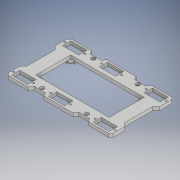
# Autodesk Inventor part: BODY_TOP
Saved by Autodesk Inventor 2017.3 (Build 213256000, 256)
## iProperties
Created: 2017-09-24
Part Number: BODY_TOP
Material: Generic
Document SubType Name: Modeling
Designer: Alexander Miller
Density: 1 g/cm^3
Appearance: Default
body_C_Top: 5,000 mm
Author: Alexander Miller
Autodesk Inventor part; units mm, degrees
ref_plane "YZ Plane" through (0, 0, 0) normal (1, 0, 0) x (0, 1, 0)
ref_plane "XZ Plane" through (0, 0, 0) normal (0, 1, 0) x (-1, 0, 0)
ref_plane "XY Plane" through (0, 0, 0) normal (0, 0, 1) x (1, 0, 0)
sketch "Sketch1" plane through (0, 0, 0) normal (0, 1, 0) x (-1, 0, 0)
  line L0 (45, -75) -> (-45, -75)
  line L1 (-45, -75) -> (-45, 75)
  line L2 (-45, 75) -> (45, 75)
  line L3 (45, 75) -> (45, -75)
  point P0 (0, 0)
  point P1 (0, -75)
  point P2 (45, 0)
  dimension "d0" = 90
  dimension "d1" = 150
  constraints: 8 end point, 2 midpoint, 2 parallel, 1 horizontal, 1 horizontal alignment, 1 perpendicular, 1 vertical alignment
  measures "d0" distance of L0.start L0.end
  measures "d1" distance of L2.end L0.start
extrude "Extrusion1" add sketch "Sketch1" along normal blind 5
sketch "Sketch2" plane through (0, 5, 0) normal (0, 1, 0) x (1, 0, 0)
  line L0 (-42.5, 69.75) -> (-30.5, 69.75)
  line L1 (-30.5, 69.75) -> (-30.5, 46.75)
  line L2 (-30.5, 46.75) -> (-42.5, 46.75)
  line L3 (-42.5, 46.75) -> (-42.5, 69.75)
  line L4 (-42.5, 17) -> (-30.5, 17)
  line L5 (-30.5, 17) -> (-30.5, -6)
  line L6 (-30.5, -6) -> (-42.5, -6)
  line L7 (-42.5, -6) -> (-42.5, 17)
  line L8 (-42.5, -46.75) -> (-30.5, -46.75)
  line L9 (-30.5, -46.75) -> (-30.5, -69.75)
  line L10 (-30.5, -69.75) -> (-42.5, -69.75)
  line L11 (-42.5, -69.75) -> (-42.5, -46.75)
  line L12 (-45, 75) -> (-45, -75) projected
  line L13 (45, 75) -> (-45, 75) projected
  line L14 (-45, -75) -> (45, -75) projected
  circle A0 centre (-36.5, 0) radius 6 construction
  circle A1 centre (-36.5, 72.5) radius 1.25
  circle A2 centre (-36.5, 44) radius 1.25
  circle A3 centre (-36.5, 19.75) radius 1.25
  circle A4 centre (-36.5, -8.75) radius 1.25
  circle A5 centre (-36.5, -44) radius 1.25
  circle A6 centre (-36.5, -72.5) radius 1.25
  line L15 (0, 105) -> (0, -105) construction
  line L16 (42.5, 69.75) -> (30.5, 69.75)
  line L17 (30.5, 69.75) -> (30.5, 46.75)
  line L18 (30.5, 46.75) -> (42.5, 46.75)
  line L19 (42.5, 46.75) -> (42.5, 69.75)
  line L20 (42.5, 17) -> (30.5, 17)
  line L21 (30.5, 17) -> (30.5, -6)
  line L22 (30.5, -6) -> (42.5, -6)
  line L23 (42.5, -6) -> (42.5, 17)
  line L24 (42.5, -46.75) -> (30.5, -46.75)
  line L25 (30.5, -46.75) -> (30.5, -69.75)
  line L26 (30.5, -69.75) -> (42.5, -69.75)
  line L27 (42.5, -69.75) -> (42.5, -46.75)
  circle A7 centre (36.5, 72.5) radius 1.25
  circle A8 centre (36.5, 44) radius 1.25
  circle A9 centre (36.5, 19.75) radius 1.25
  circle A10 centre (36.5, -8.75) radius 1.25
  circle A11 centre (36.5, -44) radius 1.25
  circle A12 centre (36.5, -72.5) radius 1.25
  point P0 (0, 0)
  point P1 (-36.5, 46.75)
  point P2 (-36.5, 17)
  point P3 (-36.5, -6)
  point P4 (-36.5, -46.75)
  point P5 (-36.5, 69.75)
  point P6 (-36.5, -69.75)
  dimension "d4" = 2.5
  dimension "d5" = 5.25
  dimension "d6" = 23
  dimension "d7" = 12
  dimension "d8" = 5.25
  dimension "d9" = 2.5
  dimension "d10" = 1.5
  dimension "d11" = 1.5
  dimension "d12" = 1.5
  dimension "d13" = 1.5
  dimension "d14" = 1.5
  dimension "d15" = 1.5
  constraints: 48 end point, 18 symmetric about line, 13 centre point, 8 vertical alignment, 6 midpoint, 6 parallel, 5 equal radius, 3 equal length, 3 horizontal, 3 perpendicular, 3 tangent, 2 point on line, 1 horizontal alignment, 6 other
  measures "d4" distance between parallel lines of L3 L12
  measures "d5" distance between parallel lines of L13 L0
  measures "d6" distance of L2.end L0.start
  measures "d7" distance of L0.start L0.end
  measures "d8" distance between parallel lines of L14 L10
  measures "d9" diameter of A1
  measures "d10" distance edge to line of A1 L0
  measures "d11" distance edge to line of A2 L2
  measures "d12" distance edge to line of A3 L4
  measures "d13" distance edge to line of A4 L6
  measures "d14" distance edge to line of A5 L8
  measures "d15" distance edge to line of A6 L10
extrude "Extrusion2" cut sketch "Sketch2" against normal through all
sketch "Sketch3" plane through (0, 5, 0) normal (0, 1, 0) x (1, 0, 0)
  line L0 (45, 42.875) -> (40, 39.875)
  line L1 (40, 39.875) -> (40, 23.875)
  line L2 (45, -75) -> (45, 75) projected
  line L3 (40, 23.875) -> (45, 20.875)
  line L4 (45, 20.875) -> (45, 42.875)
  line L5 (42.5, 46.75) -> (30.5, 46.75) projected
  line L6 (36.5, 46.75) -> (36.5, 17) construction
  line L7 (30.5, 17) -> (42.5, 17) projected
  line L8 (-63, 0) -> (63, 0) projected
  line L9 (0, 105) -> (0, -105) projected
  line L10 (45, -42.875) -> (40, -39.875)
  line L11 (40, -39.875) -> (40, -23.875)
  line L12 (40, -23.875) -> (45, -20.875)
  line L13 (45, -20.875) -> (45, -42.875)
  line L14 (-45, 42.875) -> (-40, 39.875)
  line L15 (-40, 39.875) -> (-40, 23.875)
  line L16 (-40, 23.875) -> (-45, 20.875)
  line L17 (-45, 20.875) -> (-45, 42.875)
  line L18 (-45, -42.875) -> (-40, -39.875)
  line L19 (-40, -39.875) -> (-40, -23.875)
  line L20 (-40, -23.875) -> (-45, -20.875)
  line L21 (-45, -20.875) -> (-45, -42.875)
  line L22 (25, 75) -> (-25, 75)
  line L23 (-25, 75) -> (-20, 70)
  line L24 (-20, 70) -> (20, 70)
  line L25 (20, 70) -> (25, 75)
  line L26 (45, 75) -> (-45, 75) projected
  line L27 (25, -75) -> (-25, -75)
  line L28 (-25, -75) -> (-20, -70)
  line L29 (-20, -70) -> (20, -70)
  line L30 (20, -70) -> (25, -75)
  point P0 (0, 0)
  point P1 (45, 31.875)
  point P2 (40, 31.875)
  point P3 (36.5, 31.875)
  point P4 (0, 70)
  point P5 (0, 75)
  dimension "d38" = 16
  dimension "d39" = 22
  dimension "d40" = 40
  dimension "d41" = 50
  dimension "d42" = 5
  dimension "d43" = 5
  constraints: 50 end point, 16 symmetric about line, 7 midpoint, 3 parallel, 2 collinear, 2 equal length, 2 horizontal alignment, 2 vertical alignment, 1 perpendicular
  measures "d38" distance of L0.end L1.end
  measures "d39" distance of L3.end L0.start
  measures "d40" distance of L23.end L24.end
  measures "d41" distance of L22.start L22.end
  measures "d42" distance between parallel lines of L26 L24
  measures "d43" distance between parallel lines of L1 L4
extrude "Extrusion3" cut sketch "Sketch3" against normal through all contours L2 L3 L1 L0 | L2 L10 L11 L12 | L29 L30 L27 L9 | L9 L27 L28 L29 | L25 L24 L9 L22 | L9 L24 L23 L22 | L14 L15 L16 L17 | L21 L20 L19 L18
chamfer "Chamfer1" distance 3 angle 45 4 edges at (45, 2.5, 75) (-45, 2.5, 75) (-45, 2.5, -75) (45, 2.5, -75)
sketch "Sketch4" plane through (0, 5, 0) normal (0, 1, 0) x (1, 0, 0)
  line L0 (25, 52.5) -> (-25, 52.5)
  line L1 (-25, 52.5) -> (-25, -52.5)
  line L2 (-25, -52.5) -> (25, -52.5)
  line L3 (25, -52.5) -> (25, 52.5)
  point P0 (0, 0)
  point P1 (25, 0)
  point P2 (0, 52.5)
  dimension "d23" = 105
  dimension "d24" = 50
  constraints: 8 end point, 2 midpoint, 2 parallel, 1 horizontal, 1 horizontal alignment, 1 perpendicular, 1 vertical alignment
  measures "d23" distance of L2.end L0.start
  measures "d24" distance of L1.end L2.end
extrude "Extrusion4" cut sketch "Sketch4" against normal blind 5
sketch "Sketch7" plane through (0, 5, 0) normal (0, 1, 0) x (1, 0, 0)
  circle A0 centre (36.5, 31.875) radius 1.675
  line L0 (-63, 0) -> (63, 0) projected
  line L1 (0, 105) -> (0, -105) projected
  line L2 (40, 23.875) -> (40, 39.875) projected
  line L3 (30.5, 17) -> (42.5, 17) projected
  circle A1 centre (36.5, -31.875) radius 1.675
  circle A2 centre (-36.5, 31.875) radius 1.675
  circle A3 centre (-36.5, -31.875) radius 1.675
  point P0 (0, 0)
  point P1 (40, 31.875)
  point P2 (36.5, 17)
  dimension "d44" = 3.35
  constraints: 4 centre point, 3 symmetric about line, 2 midpoint, 1 horizontal alignment, 1 vertical alignment, 3 other
  measures "d44" diameter of A0
extrude "Extrusion7" cut sketch "Sketch7" against normal through all
sketch "Sketch8" plane through (0, 0, 0) normal (0, -1, 0) x (1, 0, 0)
  line L0 (-38.675, -46.175) -> (-34.325, -46.175)
  line L1 (-34.325, -46.175) -> (-34.325, -41.825)
  line L2 (-34.325, -41.825) -> (-38.675, -41.825)
  line L3 (-38.675, -41.825) -> (-38.675, -46.175)
  line L4 (-38.675, -74.675) -> (-34.325, -74.675)
  line L5 (-34.325, -74.675) -> (-34.325, -70.325)
  line L6 (-34.325, -70.325) -> (-38.675, -70.325)
  line L7 (-38.675, -70.325) -> (-38.675, -74.675)
  line L8 (-38.675, -21.925) -> (-34.325, -21.925)
  line L9 (-34.325, -21.925) -> (-34.325, -17.575)
  line L10 (-34.325, -17.575) -> (-38.675, -17.575)
  line L11 (-38.675, -17.575) -> (-38.675, -21.925)
  line L12 (-38.675, 6.575) -> (-34.325, 6.575)
  line L13 (-34.325, 6.575) -> (-34.325, 10.925)
  line L14 (-34.325, 10.925) -> (-38.675, 10.925)
  line L15 (-38.675, 10.925) -> (-38.675, 6.575)
  line L16 (-38.675, 41.825) -> (-34.325, 41.825)
  line L17 (-34.325, 41.825) -> (-34.325, 46.175)
  line L18 (-34.325, 46.175) -> (-38.675, 46.175)
  line L19 (-38.675, 46.175) -> (-38.675, 41.825)
  line L20 (-34.325, 70.325) -> (-38.675, 70.325)
  line L21 (-38.675, 70.325) -> (-38.675, 74.675)
  line L22 (-38.675, 74.675) -> (-34.325, 74.675)
  line L23 (-34.325, 74.675) -> (-34.325, 70.325)
  circle A0 centre (-36.5, -72.5) radius 1.25 projected
  circle A1 centre (-36.5, -44) radius 1.25 projected
  circle A2 centre (-36.5, -19.75) radius 1.25 projected
  circle A3 centre (-36.5, 8.75) radius 1.25 projected
  circle A4 centre (-36.5, 44) radius 1.25 projected
  circle A5 centre (-36.5, 72.5) radius 1.25 projected
  line L24 (0, -105) -> (0, 105) projected
  line L25 (38.675, -46.175) -> (34.325, -46.175)
  line L26 (34.325, -46.175) -> (34.325, -41.825)
  line L27 (34.325, -41.825) -> (38.675, -41.825)
  line L28 (38.675, -41.825) -> (38.675, -46.175)
  line L29 (38.675, -74.675) -> (34.325, -74.675)
  line L30 (34.325, -74.675) -> (34.325, -70.325)
  line L31 (34.325, -70.325) -> (38.675, -70.325)
  line L32 (38.675, -70.325) -> (38.675, -74.675)
  line L33 (38.675, -21.925) -> (34.325, -21.925)
  line L34 (34.325, -21.925) -> (34.325, -17.575)
  line L35 (34.325, -17.575) -> (38.675, -17.575)
  line L36 (38.675, -17.575) -> (38.675, -21.925)
  line L37 (38.675, 6.575) -> (34.325, 6.575)
  line L38 (34.325, 6.575) -> (34.325, 10.925)
  line L39 (34.325, 10.925) -> (38.675, 10.925)
  line L40 (38.675, 10.925) -> (38.675, 6.575)
  line L41 (38.675, 41.825) -> (34.325, 41.825)
  line L42 (34.325, 41.825) -> (34.325, 46.175)
  line L43 (34.325, 46.175) -> (38.675, 46.175)
  line L44 (38.675, 46.175) -> (38.675, 41.825)
  line L45 (34.325, 70.325) -> (38.675, 70.325)
  line L46 (38.675, 70.325) -> (38.675, 74.675)
  line L47 (38.675, 74.675) -> (34.325, 74.675)
  line L48 (34.325, 74.675) -> (34.325, 70.325)
  point P0 (0, 0)
  point P1 (-36.5, -74.675)
  point P2 (-36.5, -46.175)
  point P3 (-36.5, -41.825)
  point P4 (-36.5, -21.925)
  point P5 (-36.5, -17.575)
  point P6 (-36.5, 6.575)
  point P7 (-36.5, 10.925)
  point P8 (-36.5, 41.825)
  point P9 (-36.5, 46.175)
  point P10 (-36.5, 70.325)
  point P11 (-38.675, -72.5)
  point P12 (-38.675, -44)
  point P13 (-38.675, -19.75)
  point P14 (-38.675, 8.75)
  point P15 (-38.675, 72.5)
  point P16 (-38.675, 44)
  dimension "d47" = 4.35
  constraints: 96 end point, 24 symmetric about line, 16 midpoint, 12 parallel, 11 equal length, 6 horizontal, 6 horizontal alignment, 6 perpendicular, 6 vertical alignment, 2 point on line
  measures "d47" distance of L6.end L4.start
extrude "Extrusion8" cut sketch "Sketch8" against normal blind 1.725
sketch "Sketch9" plane through (0, 5, 0) normal (0, 1, 0) x (1, 0, 0)
  circle A0 centre (36.5, 31.875) radius 2.925
  circle A1 centre (36.5, -31.875) radius 2.925
  circle A2 centre (-36.5, -31.875) radius 2.925
  circle A3 centre (-36.5, 31.875) radius 2.925
  circle A4 centre (36.5, 31.875) radius 1.675 projected
  circle A5 centre (36.5, -31.875) radius 1.675 projected
  circle A6 centre (-36.5, -31.875) radius 1.675 projected
  circle A7 centre (-36.5, 31.875) radius 1.675 projected
  point P0 (0, 0)
  dimension "d50" = 5.85
  constraints: 4 centre point, 4 concentric, 3 equal radius
  measures "d50" diameter of A0
extrude "Extrusion9" cut sketch "Sketch9" against normal blind 3
sketch "Sketch11" plane through (0, 0, 0) normal (0, -1, 0) x (1, 0, 0)
  line L0 (-19.65, -57.5) -> (-30, -57.5)
  line L1 (-30, -57.5) -> (-30, -47.15)
  line L2 (-30, -47.15) -> (-19.65, -47.15)
  line L3 (-19.65, -47.15) -> (-19.65, -57.5)
  line L4 (-30, 47.15) -> (-19.65, 47.15)
  line L5 (-19.65, 47.15) -> (-19.65, 57.5)
  line L6 (-19.65, 57.5) -> (-30, 57.5)
  line L7 (-30, 57.5) -> (-30, 47.15)
  line L8 (19.65, 57.5) -> (30, 57.5)
  line L9 (30, 57.5) -> (30, 47.15)
  line L10 (30, 47.15) -> (19.65, 47.15)
  line L11 (19.65, 47.15) -> (19.65, 57.5)
  line L12 (19.65, -57.5) -> (30, -57.5)
  line L13 (30, -57.5) -> (30, -47.15)
  line L14 (30, -47.15) -> (19.65, -47.15)
  line L15 (19.65, -47.15) -> (19.65, -57.5)
  line L16 (-25, -52.5) -> (-25, 52.5) projected
  line L17 (25, -52.5) -> (-25, -52.5) projected
  line L18 (-25, 52.5) -> (25, 52.5) projected
  line L19 (25, 52.5) -> (25, -52.5) projected
  point P0 (0, 0)
  point P1 (-19.65, -52.325)
  point P2 (19.65, -52.325)
  point P3 (-19.65, 52.325)
  point P4 (19.65, 52.325)
  point P5 (-24.825, -47.15)
  point P6 (-24.825, 47.15)
  point P7 (24.825, 47.15)
  point P8 (24.825, -47.15)
  dimension "d60" = 5.35
  dimension "d61" = 5.35
  dimension "d62" = 5.35
  dimension "d63" = 5.35
  dimension "d64" = 5
  dimension "d65" = 5
  constraints: 32 end point, 8 midpoint, 8 parallel, 6 equal length, 4 horizontal, 4 perpendicular, 2 horizontal alignment, 2 vertical alignment
  measures "d60" distance between parallel lines of L3 L16
  measures "d61" distance between parallel lines of L17 L2
  measures "d62" distance between parallel lines of L18 L4
  measures "d63" distance between parallel lines of L19 L15
  measures "d64" distance between parallel lines of L0 L17
  measures "d65" distance between parallel lines of L16 L1
extrude "Extrusion11" add sketch "Sketch11" along normal blind 4.35 contours L0 L1 L2 L16 L17 L3 | L17 L16 L2 L3 | L17 L19 L14 L13 L12 L15 | L15 L14 L19 L17 | L16 L18 L5 L4 | L4 L7 L6 L5 L18 L16 | L19 L18 L11 L8 L9 L10 | L10 L11 L18 L19
chamfer "Chamfer2" distance 4.35 angle 45 8 edges at (-24.825, -4.35, 57.5) (-30, -4.35, 52.325) (24.825, -4.35, 57.5) (30, -4.35, 52.325) (-30, -4.35, -52.325) (-24.825, -4.35, -57.5) (30, -4.35, -52.325) (24.825, -4.35, -57.5)
sketch "Sketch13" plane through (0, -4.35, 0) normal (0, -1, 0) x (1, 0, 0)
  line L0 (-25.65, -53.15) -> (-25.65, -47.15) projected
  line L1 (-19.65, -53.15) -> (-25.65, -53.15) projected
  line L2 (-19.65, -53.15) -> (-19.65, -47.15) projected
  line L3 (-19.65, -47.15) -> (-25.65, -47.15) projected
  line L4 (25.65, -47.15) -> (25.65, -53.15) projected
  line L5 (25.65, -47.15) -> (19.65, -47.15) projected
  line L6 (19.65, -47.15) -> (19.65, -53.15) projected
  line L7 (25.65, -53.15) -> (19.65, -53.15) projected
  line L8 (25.65, 53.15) -> (25.65, 47.15) projected
  line L9 (19.65, 53.15) -> (25.65, 53.15) projected
  line L10 (19.65, 53.15) -> (19.65, 47.15) projected
  line L11 (19.65, 47.15) -> (25.65, 47.15) projected
  line L12 (-25.65, 53.15) -> (-19.65, 53.15) projected
  line L13 (-25.65, 47.15) -> (-25.65, 53.15) projected
  line L14 (-25.65, 47.15) -> (-19.65, 47.15) projected
  line L15 (-19.65, 47.15) -> (-19.65, 53.15) projected
  point P0 (0, 0)
extrude "Extrusion12" cut sketch "Sketch13" against normal blind 3.35
equation "\"d0\" = body_B"
equation "\"d1\" = body_A"
equation "\"d2\" = body_C_Top"
equation "\"d4\" = 0.5 * body_C"
equation "\"d6\" = servo_A"
equation "\"d7\" = servo_B"
equation "\"d8\" = d5"
equation "\"d9\" = servo_H"
equation "\"d10\" = servo_L"
equation "\"d11\" = d10"
equation "\"d12\" = d10"
equation "\"d13\" = d10"
equation "\"d14\" = d10"
equation "\"d15\" = d10"
equation "\"d16\" = body_C"
equation "\"d29\" = body_C"
equation "\"d44\" = nut_C"
equation "\"d47\" = nut_A_1"
equation "\"d48\" = nut_B_1"
equation "\"d50\" = screw_m3_C"
equation "\"d60\" = magnet_A"
equation "\"d61\" = magnet_A"
equation "\"d62\" = magnet_A"
equation "\"d63\" = magnet_A"
equation "\"d71\" = magnet_B"
equation "\"body_C_Top\" = body_C"
equation "\"body_B\" = 90"
equation "\"body_A\" = 150"
equation "\"body_C\" = 5"
equation "\"servo_A\" = 23"
equation "\"servo_B\" = 12"
equation "\"servo_H\" = 2.5"
equation "\"servo_L\" = 1.5"
equation "\"nut_C\" = 3.35"
equation "\"nut_A_1\" = 4.35"
equation "\"nut_B_1\" = 1.725"
equation "\"screw_m3_C\" = 5.85"
equation "\"magnet_A\" = 5.35"
equation "\"magnet_B\" = 3.35"
body "Solid1"
